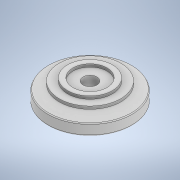
# Autodesk Inventor part: pulley
Saved by Autodesk Inventor 2022 (Build 260153000, 153)
## iProperties
Created: 2022-02-28
Part Number: pulley
Material: Generic
Document SubType Name: Modeling
Designer: Frey
Density: 1 g/cm^3
Appearance: Default
Author: Frey
Autodesk Inventor part; units mm, degrees
ref_plane "YZ Plane" through (0, 0, 0) normal (1, 0, 0) x (0, 1, 0)
ref_plane "XZ Plane" through (0, 0, 0) normal (0, 1, 0) x (-1, 0, 0)
ref_plane "XY Plane" through (0, 0, 0) normal (0, 0, 1) x (1, 0, 0)
sketch "Sketch1" plane through (0, 0, 0) normal (0, 0, 1) x (1, 0, 0)
  line L0 (0, 0) -> (-15, 0)
  line L1 (-15, 0) -> (-15, 4)
  line L2 (-15, 4) -> (-11, 5.6)
  line L3 (-11, 5.6) -> (-11, 6.6)
  line L4 (-11, 6.6) -> (0, 6.6)
  line L5 (0, 6.6) -> (0, 0)
  dimension "d1" = 4
  dimension "d5" = 1
  dimension "d12" = 11
  dimension "d13" = 2.6
  dimension "d14" = 4
  constraints: 12 end point, 2 perpendicular, 1 horizontal, 1 parallel
  measures "d1" distance of L0.end L1.end
  measures "d5" distance of L2.end L3.end
  measures "d12" distance between parallel lines of L3 L5
  measures "d13" vertical distance of L3.end L1.end
  measures "d14" distance between parallel lines of L3 L1
revolve "Revolution1" add sketch "Sketch1" angle 360 about axis through (0, 6.6, 0) along (0, -1, 0)
fillet "Fillet1" radius 0.5 1 edges at (15, 0, 0)
sketch "Sketch3" plane through (0, 0, 0) normal (0, -1, 0) x (1, 0, 0)
  circle A0 centre (0, 0) radius 2.5
  dimension "d15" = 5
  constraints: 1 centre point, 1 coincident
  measures "d15" diameter of A0
extrude "Extrusion2" cut sketch "Sketch3" against normal up to surface (6.6 mm away)
fillet "Fillet2" radius 0.4 1 edges at (15, 4, 0)
sketch "Sketch4" plane through (0, 6.6, 0) normal (0, 1, 0) x (1, 0, 0)
  circle A0 centre (0, 0) radius 8
  circle A1 centre (0, 0) radius 6.1
  dimension "d19" = 16
  dimension "d20" = 1.9
  constraints: 2 centre point, 2 coincident
  measures "d19" diameter of A0
  measures "d20" radial gap between concentric circles of A0 A1
extrude "Extrusion3" add sketch "Sketch4" along normal blind 1
body "Solid1"
